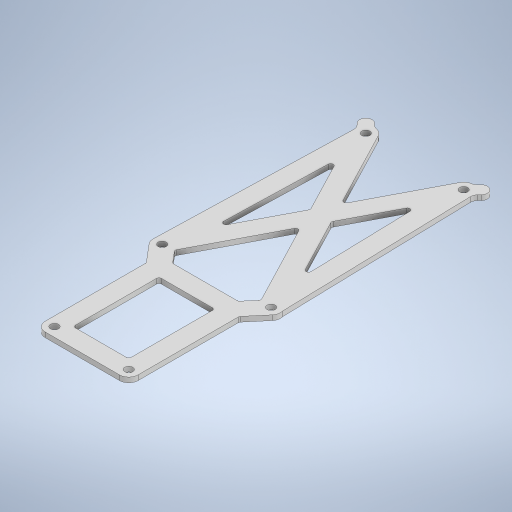
# Autodesk Inventor part: mocowanie
Saved by Autodesk Inventor 2023 (Build 270158000, 158)
## iProperties
Created: 2024-05-17
Part Number: mocowanie
Material: Ogólny
Document SubType Name: Modeling
Designer: kamil
Density: 1 g/cm^3
Appearance: Domyślna
Author: kamil
Autodesk Inventor part; units mm, degrees
ref_plane "YZ Plane" through (0, 0, 0) normal (1, 0, 0) x (0, 1, 0)
ref_plane "XZ Plane" through (0, 0, 0) normal (0, 1, 0) x (-1, 0, 0)
ref_plane "XY Plane" through (0, 0, 0) normal (0, 0, 1) x (1, 0, 0)
sketch "Szkic1" plane through (0, 0, 0) normal (0, 1, 0) x (-1, 0, 0)
  line L0 (-14.9332, 17.4281) -> (15.0668, 17.4281) construction
  line L1 (-14.9332, 13.6781) -> (15.0668, 13.6781)
  line L2 (15.0668, 21.1781) -> (-14.9332, 21.1781)
  arc A0 (-14.9332, 21.1781) -> (-14.9332, 13.6781) centre (-14.9332, 17.4281) ccw
  arc A1 (15.0668, 13.6781) -> (15.0668, 21.1781) centre (15.0668, 17.4281) ccw
  line L3 (0.0668, 17.4281) -> (0.0668, -37.9617) construction
  line L4 (15.0668, 17.4281) -> (15.0668, -55.6314) construction
  line L5 (-14.9332, 17.4281) -> (-14.9332, -55.6314) construction
  line L6 (22.0668, -33.0639) -> (15.0668, -24.7796) construction
  line L7 (24.9311, -30.6436) -> (17.9311, -22.3593)
  line L8 (12.2024, -27.1999) -> (19.2024, -35.4842)
  arc A2 (19.2024, -35.4842) -> (24.9311, -30.6436) centre (22.0668, -33.0639) ccw
  arc A3 (17.9311, -22.3593) -> (12.2024, -27.1999) centre (15.0668, -24.7796) ccw
  line L9 (-21.9332, -33.0639) -> (-14.9332, -24.7796) construction
  line L10 (-19.0689, -35.4842) -> (-12.0689, -27.1999)
  line L11 (-17.7976, -22.3593) -> (-24.7976, -30.6436)
  arc A4 (-24.7976, -30.6436) -> (-19.0689, -35.4842) centre (-21.9332, -33.0639) ccw
  arc A5 (-12.0689, -27.1999) -> (-17.7976, -22.3593) centre (-14.9332, -24.7796) ccw
  line L12 (15.0668, 17.4281) -> (15.0668, -24.7796) construction
  line L13 (11.3168, 17.4281) -> (11.3168, -24.7796)
  line L14 (18.8168, -24.7796) -> (18.8168, 17.4281)
  arc A6 (18.8168, 17.4281) -> (11.3168, 17.4281) centre (15.0668, 17.4281) ccw
  arc A7 (11.3168, -24.7796) -> (18.8168, -24.7796) centre (15.0668, -24.7796) ccw
  line L15 (-14.9332, 17.4281) -> (-14.9332, -24.7796) construction
  line L16 (-18.6832, 17.4281) -> (-18.6832, -24.7796)
  line L17 (-11.1832, -24.7796) -> (-11.1832, 17.4281)
  arc A8 (-11.1832, 17.4281) -> (-18.6832, 17.4281) centre (-14.9332, 17.4281) ccw
  arc A9 (-18.6832, -24.7796) -> (-11.1832, -24.7796) centre (-14.9332, -24.7796) ccw
  line L18 (-14.9332, -24.7796) -> (15.0668, -24.7796) construction
  line L19 (-14.9332, -21.0296) -> (15.0668, -21.0296)
  line L20 (15.0668, -28.5296) -> (-14.9332, -28.5296)
  arc A10 (-14.9332, -21.0296) -> (-14.9332, -28.5296) centre (-14.9332, -24.7796) ccw
  arc A11 (15.0668, -28.5296) -> (15.0668, -21.0296) centre (15.0668, -24.7796) ccw
  line L21 (22.0668, -33.0639) -> (19.8168, -113.0323) construction
  line L22 (18.3183, -32.9584) -> (16.0683, -112.9268)
  line L23 (23.5653, -113.1377) -> (25.8153, -33.1694)
  arc A12 (25.8153, -33.1694) -> (18.3183, -32.9584) centre (22.0668, -33.0639) ccw
  arc A13 (16.0683, -112.9268) -> (23.5653, -113.1377) centre (19.8168, -113.0323) ccw
  line L24 (-21.8084, -33.1694) -> (-19.6832, -113.0323) construction
  line L25 (-25.5571, -33.2691) -> (-23.4319, -113.132)
  line L26 (-15.9346, -112.9325) -> (-18.0597, -33.0696)
  arc A14 (-18.0597, -33.0696) -> (-25.5571, -33.2691) centre (-21.8084, -33.1694) ccw
  arc A15 (-23.4319, -113.132) -> (-15.9346, -112.9325) centre (-19.6832, -113.0323) ccw
  line L27 (22.0668, -33.0639) -> (-19.6832, -113.0323) construction
  line L28 (18.7425, -31.3284) -> (-23.0075, -111.2967)
  line L29 (-16.359, -114.7678) -> (25.391, -34.7994)
  arc A16 (25.391, -34.7994) -> (18.7425, -31.3284) centre (22.0668, -33.0639) ccw
  arc A17 (-23.0075, -111.2967) -> (-16.359, -114.7678) centre (-19.6832, -113.0323) ccw
  line L30 (-21.8084, -33.1694) -> (19.8168, -113.0323) construction
  line L31 (-25.1338, -34.9026) -> (16.4914, -114.7655)
  line L32 (23.1422, -111.299) -> (-18.483, -31.4361)
  arc A18 (-18.483, -31.4361) -> (-25.1338, -34.9026) centre (-21.8084, -33.1694) ccw
  arc A19 (16.4914, -114.7655) -> (23.1422, -111.299) centre (19.8168, -113.0323) ccw
  point P0 (0, 0)
  point P1 (18.5668, -28.9217)
  point P2 (-18.4332, -28.9217)
  point P3 (15.0668, -3.6757)
  point P4 (-14.9332, -3.6757)
  point P5 (0.0668, -24.7796)
  point P6 (20.9418, -73.0481)
  point P7 (-20.7458, -73.1008)
  point P8 (1.1918, -73.0481)
  point P9 (-0.9958, -73.1008)
  point P10 (-18.6832, -23.4074)
  point P11 (-25.5347, -34.1087)
  point P12 (0.0805, -83.2794)
  point P13 (24.9311, -30.6436)
  point P14 (18.8168, -23.4074)
  point P15 (4.3129, -75.1727)
  point P16 (17.8606, -49.2232)
  point P17 (16.474, -98.5053)
  point P18 (-4.1462, -75.1698)
  point P19 (-16.319, -98.4856)
  point P20 (-17.6277, -49.3039)
  point P21 (0.0861, -67.0631)
  point P22 (-17.4016, -33.511)
  point P23 (-13.1924, -28.5296)
  point P24 (13.3259, -28.5296)
  point P25 (17.5771, -33.5607)
  point P26 (11.3168, 13.6781)
  point P27 (11.3168, -21.0296)
  point P28 (-11.1832, -21.0296)
  point P29 (-11.1832, 13.6781)
  dimension "d0" = 7.5
  dimension "d1" = 7.5
  dimension "d2" = 7.5
  dimension "d3" = 7.5
  dimension "d4" = 7.5
  dimension "d5" = 7.5
  dimension "d6" = 7.5
  constraints: 86 end point, 40 point on circle, 40 tangent, 20 centre point, 10 midpoint, 10 parallel, 3 vertical, 2 concentric, 2 perpendicular, 2 point on line, 1 collinear, 1 horizontal
  measures "d0" diameter of A1
  measures "d1" diameter of A3
  measures "d2" diameter of A5
  measures "d3" diameter of A13
  measures "d4" diameter of A15
  measures "d5" diameter of A17
  measures "d6" diameter of A19
extrude "Wyciągnięcie proste1" add sketch "Szkic1" along normal blind 2 contours A0 A8 L17 L1 | L1 L17 L19 A5 L11 L16 A0 | L17 A8 L2 A6 L13 L1 | L13 A6 A1 L1 | L1 A1 L14 L7 A3 L19 L13 | L19 L13 A3 L8 L20 L10 A5 L17 | L17 A5 L19 | L16 A9 L20 L10 L32 A14 L25 A4 L11 | L11 A10 L16 | L19 A3 L13 | A5 A9 A10 | A3 A11 A7 | L10 L20 A9 | L25 A18 L31 A4 | A4 L31 L26 L28 A17 L25 | L14 A11 L7 | L7 A12 L28 L8 L20 A7 L14 | A7 L20 L8 | L31 A18 A14 L26 L10 A4 | A4 L10 L26 L31 | A17 L28 L26 A15 | A2 L8 L22 A12 | L32 L28 L31 L26 L10 | L10 L26 A14 L32 | A15 L26 L28 L31 L29 | L23 A19 L32 L22 L29 A2 | A12 L22 L8 L28 | L8 L22 L29 L32 L28 | L32 L29 L31 L28 | L29 L32 L22 A13 L31 | L29 L22 L8 A2 | A13 L22 L32 A19
fillet "Zaokrąglenie1" radius 1 18 edges at (-0.0805, 1, -83.2794) (-4.3129, 1, -75.1727) (4.1462, 1, -75.1698) (-0.0861, 1, -67.0631) (-17.8606, 1, -49.2232) (-16.474, 1, -98.5053) (16.319, 1, -98.4856) (17.6277, 1, -49.3039) (17.4016, 1, -33.511) (13.1924, 1, -28.5296) (-18.8168, 1, -23.4074) (-17.5771, 1, -33.5607) (-13.3259, 1, -28.5296) (-11.3168, 1, -21.0296) (11.1832, 1, -21.0296) (11.1832, 1, 13.6781) (-11.3168, 1, 13.6781) (18.6832, 1, -23.4074)
sketch "Szkic5" plane through (0, 0, 0) normal (0, -1, 0) x (1, 0, 0)
  arc A0 (18.6832, 17.4281) -> (14.9332, 21.1781) centre (14.9332, 17.4281) ccw projected
  arc A1 (-15.0668, 21.1781) -> (-18.8168, 17.4281) centre (-15.0668, 17.4281) ccw projected
  arc A2 (25.5347, -34.1087) -> (24.7976, -30.6436) centre (21.9332, -33.0639) ccw projected
  arc A3 (-24.9311, -30.6436) -> (-25.8153, -33.1694) centre (-22.0668, -33.0639) ccw projected
  arc A4 (16.359, -114.7678) -> (23.4319, -113.132) centre (19.6832, -113.0323) ccw projected
  arc A5 (-23.5653, -113.1377) -> (-16.4914, -114.7655) centre (-19.8168, -113.0323) ccw projected
  point P0 (0, 0)
hole "Otwór2" at (21.9332, 0, -33.0639) at (-22.0668, 0, -33.0639) at (14.9332, 0, 17.4281) at (-15.0668, 0, 17.4281) at (19.6832, 0, -113.0323) at (-19.8168, 0, -113.0323) direction (0, 1, 0) diameter 3.2 depth 6
sketch "Szkic6" plane through (0, 0, 0) normal (0, -1, 0) x (1, 0, 0)
  circle A0 centre (19.6832, -113.0323) radius 1.6 projected
  circle A1 centre (-19.8168, -113.0323) radius 1.6 projected
  line L0 (19.6832, -113.0323) -> (23.2188, -116.5678) construction
  line L1 (17.9155, -114.8) -> (21.451, -118.3356)
  line L2 (24.9865, -114.8) -> (21.451, -111.2645)
  arc A2 (21.451, -111.2645) -> (17.9155, -114.8) centre (19.6832, -113.0323) ccw
  arc A3 (21.451, -118.3356) -> (24.9865, -114.8) centre (23.2188, -116.5678) ccw
  line L3 (-19.8168, -113.0323) -> (-23.3523, -116.5678) construction
  line L4 (-21.5845, -111.2645) -> (-25.1201, -114.8)
  line L5 (-21.5845, -118.3356) -> (-18.049, -114.8)
  arc A4 (-18.049, -114.8) -> (-21.5845, -111.2645) centre (-19.8168, -113.0323) ccw
  arc A5 (-25.1201, -114.8) -> (-21.5845, -118.3356) centre (-23.3523, -116.5678) ccw
  line L6 (12.7282, -28.5296) -> (-12.8617, -28.5296) projected
  point P0 (0, 0)
  point P1 (21.451, -114.8)
  point P2 (-21.5845, -114.8)
  dimension "d29" = 5
  dimension "d30" = 5
  dimension "d31" = 5
  dimension "d32" = 5
  dimension "d33" = 45
  constraints: 16 end point, 8 point on circle, 8 tangent, 4 centre point, 2 midpoint, 2 parallel, 1 horizontal alignment
  measures "d29" distance of L0.start L0.end
  measures "d30" diameter of A3
  measures "d31" distance of L3.start L3.end
  measures "d32" diameter of A5
  measures "d33" angle of L6 L0
extrude "Wyciągnięcie proste3" add sketch "Szkic6" against normal blind 2
fillet "Zaokrąglenie3" radius 3 4 edges at (19.8919, 1, -116.7764) (23.4274, 1, -113.2409) (-20.0254, 1, -116.7764) (-23.561, 1, -113.2409)
